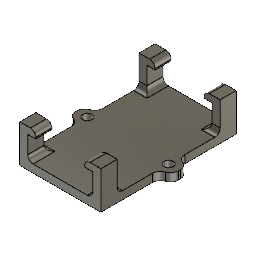
ESCClip (Autodesk Fusion 360 design; units mm, degrees)
Autodesk Fusion 360 part; units mm, degrees
note: some values were not read from the file. Chosen so that the rebuilt part matches the saved one: which pieces of a blend or face edit are solid.
sketch "Sketch1" plane through (0, 0, 0) normal (0, 0, 1) x (1, 0, 0)
  line L0 (15, 25) -> (-15, 25)
  line L1 (-15, 25) -> (-15, -25)
  line L2 (-15, -25) -> (15, -25)
  line L3 (15, -25) -> (15, 25)
  line L4 (15, 25) -> (-15, -25) construction
  line L5 (-15, 25) -> (15, -25) construction
  dimension "d1" = 30
  dimension "d2" = 50
  constraint horizontal L0
  constraint perpendicular L0 L1
  constraint parallel L0 L2
  constraint parallel L1 L3
  constraint coincident L4 origin
  constraint coincident L5 origin
  measures "d1" distance of L0.start L0.end
  measures "d2" distance of L0.start L2.end
extrude "Extrude1" add sketch "Sketch1" along normal blind 14
sketch "Sketch2" plane through (0, -25, 0) normal (0, -1, 0) x (1, 0, 0)
  line L0 (-15, 0) -> (15, 0)
  line L1 (15, 0) -> (15, 14)
  line L2 (15, 14) -> (-15, 14)
  line L3 (-15, 14) -> (-15, 0)
  line L4 (-9, 14) -> (9, 14)
  line L5 (9, 11.5) -> (12, 11.5)
  line L6 (12, 11.5) -> (12, 3)
  line L7 (12, 3) -> (-12, 3)
  line L8 (-12, 3) -> (-12, 11.5)
  line L9 (-12, 11.5) -> (-9, 11.5)
  line L10 (-9, 11.5) -> (-9, 14)
  line L11 (9, 14) -> (9, 11.5)
  dimension "d5" = 2.5
  dimension "d6" = 3
  dimension "d7" = 3
  dimension "d8" = 3
  dimension "d9" = 3
  constraint coincident L2 L4.start
  constraint coincident L2 L4.end
  constraint perpendicular L3 L4
  constraint perpendicular L3 L5
  constraint perpendicular L5 L6
  constraint perpendicular L6 L7
  constraint perpendicular L7 L8
  constraint perpendicular L8 L9
  constraint perpendicular L5 L11
  constraint equal L10 L11
  constraint equal L5 L9
  constraint equal L6 L8
  measures "d5" distance of L4.start L9.end
  measures "d6" distance of L0 L7
  measures "d7" distance of L3 L8
  measures "d8" distance of L8.end L9.end
  measures "d9" distance of L1 L6
extrude "Extrude2" cut sketch "Sketch2" against normal through all contours L2 L4 L5 L6 L7 L8 L9 L10 L11
sketch "Sketch3" plane through (15, 0, 0) normal (1, 0, 0) x (0, 1, 0)
  line L0 (-25, 0) -> (25, 0)
  line L1 (25, 0) -> (25, 14)
  line L2 (25, 14) -> (-25, 14)
  line L3 (-25, 14) -> (-25, 0)
  line L4 (-19, 14) -> (19, 14)
  line L5 (19, 14) -> (19, 3)
  line L6 (19, 3) -> (-19, 3)
  line L7 (-19, 3) -> (-19, 14)
  dimension "d11" = 6
  dimension "d12" = 6
  dimension "d13" = 3
  constraint horizontal L4
  constraint vertical L5
  constraint horizontal L6
  constraint vertical L7
  constraint coincident L2 L4.start
  measures "d11" distance of L3 L7
  measures "d12" distance of L1 L5
  measures "d13" distance of L0 L6
extrude "Extrude3" cut sketch "Sketch3" against normal through all contours L2 L4 L5 L6 L7
fillet "Fillet1" radius 2 8 edges at (13.5, -19, 3) (12, -22, 3) (-13.5, -19, 3) (-12, -22, 3) (-12, 22, 3) (12, 22, 3) (-13.5, 19, 3) (13.5, 19, 3)
fillet "Fillet1" radius 2 4 edges at (-9, 22, 14) (9, 22, 14) (9, -22, 14) (-9, -22, 14)
sketch "Sketch5" plane through (0, 0, 3) normal (0, 0, 1) x (-1, 0, 0)
  line L0 (-10, -17) -> (-10, -25)
  line L1 (-10, -25) -> (10, -25)
  line L2 (10, -25) -> (10, -17)
  line L3 (10, -17) -> (15, -17)
  line L4 (15, -17) -> (15, 17)
  line L5 (15, 17) -> (10, 17)
  line L6 (10, 17) -> (10, 25)
  line L7 (10, 25) -> (-10, 25)
  line L8 (-10, 25) -> (-10, 17)
  line L9 (-10, 17) -> (-15, 17)
  line L10 (-15, 17) -> (-15, -17)
  line L11 (-15, -17) -> (-10, -17)
  line L12 (15, -3) -> (19, -3)
  line L13 (19, -3) -> (19, 3)
  line L14 (19, 3) -> (15, 3)
  line L15 (15, 3) -> (15, -3)
  line L16 (-15, -3) -> (-19, -3)
  line L17 (-19, -3) -> (-19, 3)
  line L18 (-19, 3) -> (-15, 3)
  line L19 (-15, 3) -> (-15, -3)
  point P0 (-15, 0)
  dimension "d22" = 4
  dimension "d23" = 6
  constraint horizontal L12
  constraint vertical L13
  constraint horizontal L14
  constraint vertical L15
  constraint coincident L4 L12.start
  constraint horizontal L16
  constraint vertical L17
  constraint horizontal L18
  constraint vertical L19
  constraint coincident L10 L16.start
  constraint equal L13 L17
  constraint equal L12 L16
  constraint midpoint L19 P0
  constraint horizontal origin P0
  constraint collinear L12 L16
  measures "d22" distance of L12.start L12.end
  measures "d23" distance of L12.end L13.end
extrude "Extrude4" add sketch "Sketch5" against normal blind 3 contours L10 L16 L17 L18 L19 | L4 L12 L13 L14 L15
fillet "Fillet2" radius 3 8 edges at (-15, 3, 1.5) (-19, 3, 1.5) (-19, -3, 1.5) (-15, -3, 1.5) (15, -3, 1.5) (19, -3, 1.5) (19, 3, 1.5) (15, 3, 1.5)
sketch "Sketch6" plane through (0, 0, 3) normal (0, 0, 1) x (-1, 0, 0)
  arc A0 (-19, -0.3431) -> (-17, -3.1716) centre (-16, -0.3431) ccw
  arc A1 (-15, -6) -> (-17, -3.1716) centre (-18, -6) ccw
  line L0 (-15, -6) -> (-15, -17)
  line L1 (-15, -17) -> (-10, -17)
  line L2 (-10, -17) -> (-10, -25)
  line L3 (-10, -25) -> (10, -25)
  line L4 (10, -25) -> (10, -17)
  line L5 (10, -17) -> (15, -17)
  line L6 (15, -17) -> (15, -5.6569)
  arc A2 (17, -2.8284) -> (15, -5.6569) centre (18, -5.6569) ccw
  arc A3 (17, -2.8284) -> (19, 0) centre (16, 0) ccw
  line L7 (19, 0) -> (19, 0.3431)
  arc A4 (19, 0.3431) -> (17, 3.1716) centre (16, 0.3431) ccw
  arc A5 (15, 6) -> (17, 3.1716) centre (18, 6) ccw
  line L8 (15, 6) -> (15, 17)
  line L9 (15, 17) -> (10, 17)
  line L10 (10, 17) -> (10, 25)
  line L11 (10, 25) -> (-10, 25)
  line L12 (-10, 25) -> (-10, 17)
  line L13 (-10, 17) -> (-15, 17)
  line L14 (-15, 17) -> (-15, 6)
  arc A6 (-17, 3.1716) -> (-15, 6) centre (-18, 6) ccw
  arc A7 (-17, 3.1716) -> (-19, 0.3431) centre (-16, 0.3431) ccw
  line L15 (-19, 0.3431) -> (-19, -0.3431)
  point P0 (15, 0)
  point P1 (-15, 0)
  dimension "d27" = 4
  dimension "d28" = 4
  constraint horizontal origin P0
  constraint horizontal origin P1
  measures "d27" distance of A3.end P0
  measures "d28" distance of L15 P1
hole "Hole2" at (-15, 0, 3) at (15, 0, 3) direction (0, 0, -1) diameter 3.4 depth 13 tip angle 118
equation "d9 = d7"
equation "d12 = d11"
equation "d28 = d27"
